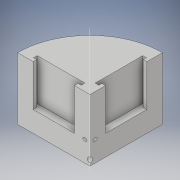
# Autodesk Inventor part: Ecke
Saved by Autodesk Inventor 2019 (Build 230136000, 136)
## iProperties
Created: 2018-08-11
Part Number: Ecke
Material: Generic
Document SubType Name: Modeling
Designer: Julia
Density: 1 g/cm^3
Appearance: Default
Author: Julia
Autodesk Inventor part; units mm, degrees
ref_plane "YZ Plane" through (0, 0, 0) normal (1, 0, 0) x (0, 1, 0)
ref_plane "XZ Plane" through (0, 0, 0) normal (0, 1, 0) x (-1, 0, 0)
ref_plane "XY Plane" through (0, 0, 0) normal (0, 0, 1) x (1, 0, 0)
sketch "Sketch1" plane through (0, 0, 0) normal (0, 1, 0) x (-1, 0, 0)
  line L0 (0, 0) -> (70, 0)
  line L1 (0, 0) -> (0, -70)
  arc A0 (0, -70) -> (70, 0) centre (0, 0) ccw
  dimension "d0" = 70
  dimension "d1" = 70
  dimension "d3" = 70
  constraints: 4 end point, 2 point on circle, 1 centre point, 1 horizontal, 1 vertical
  measures "d0" distance of L0.start L0.end
  measures "d1" distance of L0.start L1.end
  measures "d3" radius of A0
extrude "Extrusion1" add sketch "Sketch1" along normal blind 60
sketch "Sketch2" plane through (0, 0, 0) normal (1, 0, 0) x (0, 0, -1)
  line L0 (15, 60) -> (55, 60)
  line L1 (55, 60) -> (55, 20)
  line L2 (55, 20) -> (15, 20)
  line L3 (15, 20) -> (15, 60)
  line L4 (0, 60) -> (70, 60) projected
  line L5 (0, 0) -> (0, 60) projected
  dimension "d8" = 40
  dimension "d9" = 40
  dimension "d10" = 15
  constraints: 8 end point, 2 collinear, 2 parallel, 1 horizontal, 1 perpendicular
  measures "d8" distance between parallel lines of L0 L2
  measures "d9" distance between parallel lines of L1 L3
  measures "d10" distance between parallel lines of L3 L5
extrude "Extrusion2" cut sketch "Sketch2" against normal blind 7
sketch "Sketch3" plane through (-70, 0, 0) normal (0, 0, 1) x (1, 0, 0)
  line L0 (15, 60) -> (55, 60)
  line L1 (55, 60) -> (55, 20)
  line L2 (55, 20) -> (15, 20)
  line L3 (15, 20) -> (15, 60)
  line L4 (0, 60) -> (70, 60) projected
  line L5 (0, 0) -> (0, 60) projected
  point P0 (70, 0)
  point P1 (35, 20)
  point P2 (35, 60)
  dimension "d11" = 40
  dimension "d13" = 40
  dimension "d31" = 15
  constraints: 8 end point, 2 midpoint, 2 parallel, 1 collinear, 1 horizontal, 1 perpendicular, 1 vertical alignment
  measures "d11" distance between parallel lines of L1 L3
  measures "d13" distance of L0.end L1.end
  measures "d31" distance between parallel lines of L3 L5
extrude "Extrusion3" cut sketch "Sketch3" against normal blind 7
sketch "Sketch4" plane through (0, 20, -55) normal (0, 0, 1) x (1, 0, 0)
  line L0 (-3.5, 40) -> (-7, 40)
  line L1 (-7, 40) -> (-7, 0)
  line L2 (-7, 0) -> (-3.5, 0)
  line L3 (-3.5, 0) -> (-3.5, 40)
  line L4 (0, 40) -> (0, 0) projected
  line L5 (-7, 40) -> (0, 40) projected
  line L6 (0, 0) -> (-7, 0) projected
  line L7 (-7, 40) -> (-7, 0) projected
  point P0 (0, -20)
  dimension "d16" = 3.5
  constraints: 8 end point, 3 collinear, 2 parallel, 1 horizontal, 1 perpendicular
  measures "d16" distance between parallel lines of L3 L1
extrude "Extrusion4" cut sketch "Sketch4" against normal blind 3 contours L3 L2 L1 L0
sketch "Sketch5" plane through (0, 20, -15) normal (0, 0, -1) x (-1, 0, 0)
  line L0 (3.5, 40) -> (7, 40)
  line L1 (7, 0) -> (3.5, 0)
  line L2 (3.5, 0) -> (3.5, 40)
  line L3 (3.5, 40) -> (7, 40)
  line L4 (7, 40) -> (7, 0)
  line L5 (0, 0) -> (7, 0) projected
  line L6 (7, 0) -> (7, 40) projected
  point P0 (0, -20)
  dimension "d4" = 60
  dimension "d19" = 3.5
  constraints: 10 end point, 2 collinear, 2 parallel, 1 horizontal, 1 perpendicular
  measures "d19" distance between parallel lines of L2 L4
extrude "Extrusion5" cut sketch "Sketch5" against normal blind 3
sketch "Sketch8" plane through (-15, 20, 0) normal (-1, 0, 0) x (0, 0, 1)
  line L0 (-7, 40) -> (-3.5, 40)
  line L1 (-3.5, 40) -> (-3.5, 0)
  line L2 (-3.5, 0) -> (-7, 0)
  line L3 (-7, 0) -> (-7, 40)
  line L4 (-7, 40) -> (0, 40) projected
  line L5 (-7, 40) -> (-7, 0) projected
  line L6 (0, 0) -> (-7, 0) projected
  point P0 (0, -20)
  dimension "d28" = 3.5
  constraints: 8 end point, 3 collinear, 2 parallel, 1 horizontal, 1 perpendicular
  measures "d28" distance between parallel lines of L1 L3
extrude "Extrusion8" cut sketch "Sketch8" against normal blind 3
sketch "Sketch9" plane through (-55, 20, 0) normal (1, 0, 0) x (0, 0, -1)
  line L0 (3.5, 40) -> (7, 40)
  line L1 (7, 40) -> (7, 0)
  line L2 (7, 0) -> (3.5, 0)
  line L3 (3.5, 0) -> (3.5, 40)
  line L4 (0, 40) -> (7, 40) projected
  line L5 (7, 0) -> (7, 40) projected
  line L6 (0, 0) -> (7, 0) projected
  point P0 (0, -20)
  dimension "d32" = 3.5
  constraints: 8 end point, 3 collinear, 2 parallel, 1 horizontal, 1 perpendicular
  measures "d32" distance between parallel lines of L1 L3
extrude "Extrusion9" cut sketch "Sketch9" against normal blind 3
sketch "Sketch10" plane through (0, 0, 0) normal (1, 0, 0) x (0, 0, -1)
  line L0 (0, 0) -> (0, 60) projected
  arc A0 (0, 2.5) -> (0, 7.5) centre (0, 5) ccw
  line L1 (70, 0) -> (0, 0) projected
  line L2 (0, 7.5) -> (0, 2.5)
  dimension "d35" = 5
  dimension "d36" = 5
  constraints: 3 point on line, 2 end point, 2 point on circle, 1 centre point
  measures "d35" diameter of A0
  measures "d36" distance from line of L1 A0.centre
revolve "Revolution1" cut sketch "Sketch10" angle 360 about axis through (0, 0, 0) along (0, 1, 0)
ref_plane "Work Plane1" through (0, 60, 0) normal (0.7071, 0, -0.7071) x (0, -1, 0)
sketch "Sketch11" plane through (0, 60, 0) normal (0.7071, 0, -0.7071) x (0, -1, 0)
  circle A0 centre (40, 3.5) radius 1.5
  line L0 (52.5, 0) -> (0, 0) projected
  line L1 (60, 49.4975) -> (60, 0) projected
  dimension "d38" = 3
  dimension "d41" = 3.5
  dimension "d42" = 20
  constraints: 1 centre point
  measures "d38" diameter of A0
  measures "d41" distance from line of L0 A0.centre
  measures "d42" distance from line of L1 A0.centre
extrude "Extrusion10" cut sketch "Sketch11" along normal mid plane 10
body "Solid1"
